Autodesk Fusion 360 part; units mm, degrees
(part 4 of 11)
sketch "Sketch3 (3)" plane through (0, 0, 12.7) normal (0, 0, 1) x (-1, 0, 0)
  arc A0 (-21.5286, -62.8233) -> (-21.5337, -63.9888) centre (0, -63.5) ccw
  arc A1 (-22.9752, -65.6056) -> (-21.5337, -63.9888) centre (-23.1207, -64.0248) ccw
  line L0 (-22.9752, -65.6056) -> (-23.7685, -65.6787)
  spline S0 degree 5 poles (-23.7685, -65.6787) (-23.7824, -65.68) (-23.8102, -65.6829) (-23.8516, -65.6885) (-23.9064, -65.6983) (-23.9746, -65.7135) (-24.0423, -65.731) (-24.1099, -65.7498) (-24.1774, -65.7693) (-24.2448, -65.7894) (-24.3122, -65.81) (-24.3794, -65.8313) (-24.4464, -65.8535) (-24.5132, -65.8769) (-24.5799, -65.9013) (-24.6463, -65.9266) (-24.7126, -65.9529) (-24.7787, -65.9798) (-24.8447, -66.0074) (-24.9105, -66.0355) (-24.9762, -66.0643) (-25.0418, -66.0936) (-25.1072, -66.1236) (-25.1724, -66.1543) (-25.2375, -66.1856) (-25.3025, -66.2176) (-25.3672, -66.2502) (-25.4319, -66.2833) (-25.4964, -66.317) (-25.5607, -66.3513) (-25.6249, -66.386) (-25.6889, -66.4213) (-25.7528, -66.4572) (-25.8165, -66.4935) (-25.8801, -66.5304) (-25.9435, -66.5678) (-26.0067, -66.6057) (-26.0698, -66.6441) (-26.1328, -66.683) (-26.1955, -66.7224) (-26.2582, -66.7622) (-26.3206, -66.8026) (-26.383, -66.8433) (-26.4451, -66.8846) (-26.5071, -66.9263) (-26.5689, -66.9685) (-26.6306, -67.0111) (-26.6921, -67.0541) (-26.7535, -67.0976) (-26.8146, -67.1416) (-26.8757, -67.1859) (-26.9365, -67.2307) (-26.9972, -67.2759) (-27.0577, -67.3215) (-27.1181, -67.3676) (-27.1783, -67.414) (-27.2383, -67.4609) (-27.2981, -67.5082) (-27.3578, -67.5559) (-27.4173, -67.6039) (-27.4767, -67.6524) (-27.5358, -67.7013) (-27.5948, -67.7505) (-27.6536, -67.8002) (-27.7123, -67.8502) (-27.7708, -67.9006) (-27.8291, -67.9514) (-27.8872, -68.0026) (-27.9451, -68.0541) (-28.0029, -68.106) (-28.0605, -68.1583) (-28.1064, -68.2004) (-28.1408, -68.2322) (-28.1636, -68.2534) (-28.1751, -68.264) knots 0 0 0 0 0 0 0.01428571 0.02857143 0.04285714 0.05714286 0.07142857 0.08571429 0.1 0.11428571 0.12857143 0.14285714 0.15714286 0.17142857 0.18571429 0.2 0.21428571 0.22857143 0.24285714 0.25714286 0.27142857 0.28571429 0.3 0.31428571 0.32857143 0.34285714 0.35714286 0.37142857 0.38571429 0.4 0.41428571 0.42857143 0.44285714 0.45714286 0.47142857 0.48571429 0.5 0.51428571 0.52857143 0.54285714 0.55714286 0.57142857 0.58571429 0.6 0.61428571 0.62857143 0.64285714 0.65714286 0.67142857 0.68571429 0.7 0.71428571 0.72857143 0.74285714 0.75714286 0.77142857 0.78571429 0.8 0.81428571 0.82857143 0.84285714 0.85714286 0.87142857 0.88571429 0.9 0.91428571 0.92857143 0.94285714 0.95714286 0.97142857 0.98571429 1 1 1 1 1 1
  arc A2 (-28.1751, -68.264) -> (-27.9081, -69.6374) centre (0, -63.5) ccw
  spline S1 degree 5 poles (-27.9081, -69.6374) (-27.8935, -69.643) (-27.8644, -69.6541) (-27.8206, -69.6707) (-27.7622, -69.6925) (-27.6893, -69.7195) (-27.6163, -69.7459) (-27.5432, -69.772) (-27.4702, -69.7977) (-27.3971, -69.8229) (-27.324, -69.8478) (-27.2509, -69.8722) (-27.1777, -69.8962) (-27.1046, -69.9198) (-27.0314, -69.9429) (-26.9583, -69.9656) (-26.8851, -69.9879) (-26.8119, -70.0097) (-26.7387, -70.0312) (-26.6655, -70.0521) (-26.5923, -70.0727) (-26.5191, -70.0927) (-26.4458, -70.1124) (-26.3726, -70.1316) (-26.2994, -70.1503) (-26.2262, -70.1686) (-26.1531, -70.1864) (-26.0799, -70.2037) (-26.0067, -70.2206) (-25.9336, -70.237) (-25.8605, -70.2529) (-25.7874, -70.2684) (-25.7143, -70.2833) (-25.6412, -70.2978) (-25.5682, -70.3118) (-25.4952, -70.3253) (-25.4223, -70.3383) (-25.3493, -70.3507) (-25.2764, -70.3627) (-25.2036, -70.3742) (-25.1308, -70.3851) (-25.058, -70.3955) (-24.9853, -70.4053) (-24.9127, -70.4146) (-24.8401, -70.4234) (-24.7676, -70.4316) (-24.6951, -70.4392) (-24.6227, -70.4463) (-24.5503, -70.4528) (-24.4781, -70.4587) (-24.4059, -70.4641) (-24.3338, -70.4687) (-24.2618, -70.4727) (-24.1899, -70.4761) (-24.1181, -70.4787) (-24.0464, -70.4807) (-23.9748, -70.4822) (-23.9033, -70.483) (-23.832, -70.4832) (-23.7607, -70.4827) (-23.6896, -70.4814) (-23.6187, -70.479) (-23.548, -70.4756) (-23.4775, -70.4711) (-23.4072, -70.4657) (-23.337, -70.4596) (-23.267, -70.4529) (-23.1971, -70.4458) (-23.1274, -70.4379) (-23.058, -70.4287) (-22.9892, -70.4173) (-22.9346, -70.4058) (-22.8941, -70.3955) (-22.8673, -70.3878) (-22.854, -70.3838) knots -1 -1 -1 -1 -1 -1 -0.98571429 -0.97142857 -0.95714286 -0.94285714 -0.92857143 -0.91428571 -0.9 -0.88571429 -0.87142857 -0.85714286 -0.84285714 -0.82857143 -0.81428571 -0.8 -0.78571429 -0.77142857 -0.75714286 -0.74285714 -0.72857143 -0.71428571 -0.7 -0.68571429 -0.67142857 -0.65714286 -0.64285714 -0.62857143 -0.61428571 -0.6 -0.58571429 -0.57142857 -0.55714286 -0.54285714 -0.52857143 -0.51428571 -0.5 -0.48571429 -0.47142857 -0.45714286 -0.44285714 -0.42857143 -0.41428571 -0.4 -0.38571429 -0.37142857 -0.35714286 -0.34285714 -0.32857143 -0.31428571 -0.3 -0.28571429 -0.27142857 -0.25714286 -0.24285714 -0.22857143 -0.21428571 -0.2 -0.18571429 -0.17142857 -0.15714286 -0.14285714 -0.12857143 -0.11428571 -0.1 -0.08571429 -0.07142857 -0.05714286 -0.04285714 -0.02857143 -0.01428571 0 0 0 0 0 0
  line L1 (-22.854, -70.3838) -> (-22.091, -70.1544)
  arc A3 (-20.1488, -71.1135) -> (-22.091, -70.1544) centre (-21.6338, -71.6746) ccw
  arc A4 (-20.1488, -71.1135) -> (-19.7075, -72.1921) centre (0, -63.5) ccw
  arc A5 (-20.4205, -74.2376) -> (-19.7075, -72.1921) centre (-21.1599, -72.8328) ccw
  line L2 (-20.4205, -74.2376) -> (-21.1255, -74.6087)
  spline S2 degree 5 poles (-21.1255, -74.6087) (-21.1379, -74.6152) (-21.1624, -74.6285) (-21.1985, -74.6495) (-21.2454, -74.6795) (-21.3025, -74.7197) (-21.3585, -74.7617) (-21.4137, -74.805) (-21.4686, -74.8489) (-21.5232, -74.8932) (-21.5775, -74.938) (-21.6314, -74.9834) (-21.6849, -75.0296) (-21.7377, -75.0767) (-21.7899, -75.1248) (-21.8416, -75.1737) (-21.8928, -75.2233) (-21.9435, -75.2734) (-21.9939, -75.3242) (-22.044, -75.3754) (-22.0937, -75.4271) (-22.1431, -75.4793) (-22.192, -75.532) (-22.2405, -75.5853) (-22.2887, -75.6392) (-22.3364, -75.6936) (-22.3838, -75.7485) (-22.4308, -75.8038) (-22.4775, -75.8596) (-22.5239, -75.9159) (-22.5699, -75.9726) (-22.6155, -76.0297) (-22.6608, -76.0872) (-22.7058, -76.1452) (-22.7504, -76.2036) (-22.7946, -76.2624) (-22.8386, -76.3217) (-22.8822, -76.3813) (-22.9254, -76.4413) (-22.9684, -76.5017) (-23.011, -76.5625) (-23.0533, -76.6236) (-23.0952, -76.6852) (-23.1369, -76.7471) (-23.1782, -76.8093) (-23.2192, -76.8719) (-23.2598, -76.9349) (-23.3002, -76.9982) (-23.3402, -77.0619) (-23.3799, -77.1259) (-23.4193, -77.1902) (-23.4584, -77.2549) (-23.4972, -77.3199) (-23.5356, -77.3852) (-23.5738, -77.4508) (-23.6116, -77.5168) (-23.6491, -77.583) (-23.6863, -77.6496) (-23.7232, -77.7165) (-23.7598, -77.7837) (-23.7961, -77.8512) (-23.832, -77.919) (-23.8677, -77.9871) (-23.903, -78.0554) (-23.9381, -78.1241) (-23.9728, -78.193) (-24.0072, -78.2623) (-24.0413, -78.3318) (-24.0752, -78.4016) (-24.1087, -78.4716) (-24.1418, -78.542) (-24.1682, -78.5985) (-24.1878, -78.641) (-24.2008, -78.6693) (-24.2072, -78.6835) knots 0 0 0 0 0 0 0.01428571 0.02857143 0.04285714 0.05714286 0.07142857 0.08571429 0.1 0.11428571 0.12857143 0.14285714 0.15714286 0.17142857 0.18571429 0.2 0.21428571 0.22857143 0.24285714 0.25714286 0.27142857 0.28571429 0.3 0.31428571 0.32857143 0.34285714 0.35714286 0.37142857 0.38571429 0.4 0.41428571 0.42857143 0.44285714 0.45714286 0.47142857 0.48571429 0.5 0.51428571 0.52857143 0.54285714 0.55714286 0.57142857 0.58571429 0.6 0.61428571 0.62857143 0.64285714 0.65714286 0.67142857 0.68571429 0.7 0.71428571 0.72857143 0.74285714 0.75714286 0.77142857 0.78571429 0.8 0.81428571 0.82857143 0.84285714 0.85714286 0.87142857 0.88571429 0.9 0.91428571 0.92857143 0.94285714 0.95714286 0.97142857 0.98571429 1 1 1 1 1 1
  arc A6 (-24.2072, -78.6835) -> (-23.435, -79.8502) centre (0, -63.5) ccw
  spline S3 degree 5 poles (-23.435, -79.8502) (-23.4194, -79.8498) (-23.3882, -79.8489) (-23.3415, -79.8475) (-23.2792, -79.8453) (-23.2015, -79.8422) (-23.1239, -79.8388) (-23.0464, -79.8349) (-22.9691, -79.8307) (-22.8919, -79.8261) (-22.8149, -79.821) (-22.738, -79.8156) (-22.6613, -79.8098) (-22.5846, -79.8036) (-22.5082, -79.7969) (-22.4319, -79.7899) (-22.3558, -79.7825) (-22.2798, -79.7747) (-22.204, -79.7664) (-22.1283, -79.7578) (-22.0528, -79.7488) (-21.9775, -79.7393) (-21.9023, -79.7294) (-21.8274, -79.7191) (-21.7526, -79.7084) (-21.6779, -79.6973) (-21.6035, -79.6857) (-21.5293, -79.6738) (-21.4552, -79.6614) (-21.3814, -79.6485) (-21.3077, -79.6353) (-21.2343, -79.6216) (-21.161, -79.6074) (-21.088, -79.5928) (-21.0152, -79.5778) (-20.9426, -79.5623) (-20.8702, -79.5464) (-20.7981, -79.53) (-20.7261, -79.5132) (-20.6545, -79.4959) (-20.583, -79.4781) (-20.5118, -79.4599) (-20.4409, -79.4412) (-20.3702, -79.4219) (-20.2998, -79.4022) (-20.2296, -79.3821) (-20.1598, -79.3614) (-20.0902, -79.3402) (-20.0208, -79.3186) (-19.9518, -79.2964) (-19.8831, -79.2737) (-19.8147, -79.2504) (-19.7466, -79.2266) (-19.679, -79.2021) (-19.6116, -79.1771) (-19.5446, -79.1515) (-19.4779, -79.1255) (-19.4115, -79.0989) (-19.3455, -79.0718) (-19.2798, -79.044) (-19.2147, -79.0156) (-19.15, -78.9862) (-19.086, -78.956) (-19.0226, -78.9249) (-18.9598, -78.893) (-18.8973, -78.8605) (-18.8351, -78.8276) (-18.7733, -78.7942) (-18.7119, -78.7603) (-18.6513, -78.7252) (-18.5921, -78.6883) (-18.5461, -78.6568) (-18.5126, -78.6318) (-18.4908, -78.6145) (-18.48, -78.6056) knots -1 -1 -1 -1 -1 -1 -0.98571429 -0.97142857 -0.95714286 -0.94285714 -0.92857143 -0.91428571 -0.9 -0.88571429 -0.87142857 -0.85714286 -0.84285714 -0.82857143 -0.81428571 -0.8 -0.78571429 -0.77142857 -0.75714286 -0.74285714 -0.72857143 -0.71428571 -0.7 -0.68571429 -0.67142857 -0.65714286 -0.64285714 -0.62857143 -0.61428571 -0.6 -0.58571429 -0.57142857 -0.55714286 -0.54285714 -0.52857143 -0.51428571 -0.5 -0.48571429 -0.47142857 -0.45714286 -0.44285714 -0.42857143 -0.41428571 -0.4 -0.38571429 -0.37142857 -0.35714286 -0.34285714 -0.32857143 -0.31428571 -0.3 -0.28571429 -0.27142857 -0.25714286 -0.24285714 -0.22857143 -0.21428571 -0.2 -0.18571429 -0.17142857 -0.15714286 -0.14285714 -0.12857143 -0.11428571 -0.1 -0.08571429 -0.07142857 -0.05714286 -0.04285714 -0.02857143 -0.01428571 0 0 0 0 0 0
  line L3 (-18.48, -78.6056) -> (-17.8629, -78.1017)
  arc A7 (-15.7015, -78.2445) -> (-17.8629, -78.1017) centre (-16.8587, -79.3312) ccw
  arc A8 (-15.7015, -78.2445) -> (-14.881, -79.0722) centre (0, -63.5) ccw
  arc A9 (-14.757, -81.2348) -> (-14.881, -79.0722) centre (-15.9777, -80.2199) ccw
  line L4 (-14.757, -81.2348) -> (-15.2663, -81.8475)
  spline S4 degree 5 poles (-15.2663, -81.8475) (-15.2753, -81.8582) (-15.2928, -81.8799) (-15.3181, -81.9131) (-15.35, -81.9588) (-15.3874, -82.0178) (-15.423, -82.078) (-15.4575, -82.1391) (-15.4914, -82.2007) (-15.5248, -82.2625) (-15.5579, -82.3247) (-15.5903, -82.3873) (-15.622, -82.4504) (-15.6528, -82.5142) (-15.6826, -82.5785) (-15.7117, -82.6435) (-15.74, -82.7089) (-15.7677, -82.7747) (-15.7948, -82.8408) (-15.8215, -82.9073) (-15.8476, -82.9741) (-15.8732, -83.0412) (-15.8983, -83.1087) (-15.9227, -83.1765) (-15.9466, -83.2447) (-15.9699, -83.3132) (-15.9927, -83.382) (-16.0149, -83.4512) (-16.0367, -83.5206) (-16.058, -83.5903) (-16.0788, -83.6602) (-16.0991, -83.7305) (-16.1189, -83.801) (-16.1383, -83.8718) (-16.1571, -83.9428) (-16.1755, -84.0141) (-16.1934, -84.0856) (-16.2109, -84.1574) (-16.2279, -84.2294) (-16.2445, -84.3016) (-16.2606, -84.3741) (-16.2762, -84.4468) (-16.2915, -84.5197) (-16.3062, -84.5928) (-16.3206, -84.6661) (-16.3345, -84.7396) (-16.348, -84.8134) (-16.361, -84.8873) (-16.3736, -84.9615) (-16.3858, -85.0358) (-16.3976, -85.1103) (-16.409, -85.185) (-16.4199, -85.2599) (-16.4305, -85.3349) (-16.4406, -85.4102) (-16.4503, -85.4856) (-16.4596, -85.5612) (-16.4685, -85.6369) (-16.477, -85.7128) (-16.4851, -85.7889) (-16.4927, -85.8651) (-16.5, -85.9415) (-16.5069, -86.0181) (-16.5134, -86.0948) (-16.5195, -86.1716) (-16.5252, -86.2486) (-16.5305, -86.3257) (-16.5354, -86.403) (-16.54, -86.4804) (-16.5441, -86.558) (-16.5478, -86.6357) (-16.5505, -86.6979) (-16.5524, -86.7447) (-16.5535, -86.7759) (-16.5541, -86.7915) knots 0 0 0 0 0 0 0.01428571 0.02857143 0.04285714 0.05714286 0.07142857 0.08571429 0.1 0.11428571 0.12857143 0.14285714 0.15714286 0.17142857 0.18571429 0.2 0.21428571 0.22857143 0.24285714 0.25714286 0.27142857 0.28571429 0.3 0.31428571 0.32857143 0.34285714 0.35714286 0.37142857 0.38571429 0.4 0.41428571 0.42857143 0.44285714 0.45714286 0.47142857 0.48571429 0.5 0.51428571 0.52857143 0.54285714 0.55714286 0.57142857 0.58571429 0.6 0.61428571 0.62857143 0.64285714 0.65714286 0.67142857 0.68571429 0.7 0.71428571 0.72857143 0.74285714 0.75714286 0.77142857 0.78571429 0.8 0.81428571 0.82857143 0.84285714 0.85714286 0.87142857 0.88571429 0.9 0.91428571 0.92857143 0.94285714 0.95714286 0.97142857 0.98571429 1 1 1 1 1 1
  arc A10 (-16.5541, -86.7915) -> (-15.3942, -87.5738) centre (0, -63.5) ccw
  spline S5 degree 5 poles (-15.3942, -87.5738) (-15.3799, -87.5675) (-15.3514, -87.5547) (-15.3088, -87.5355) (-15.2521, -87.5097) (-15.1815, -87.4771) (-15.1111, -87.4442) (-15.041, -87.411) (-14.9712, -87.3775) (-14.9017, -87.3437) (-14.8324, -87.3095) (-14.7635, -87.2751) (-14.6948, -87.2404) (-14.6264, -87.2053) (-14.5583, -87.1699) (-14.4905, -87.1342) (-14.423, -87.0983) (-14.3558, -87.0619) (-14.2889, -87.0253) (-14.2223, -86.9884) (-14.156, -86.9511) (-14.09, -86.9136) (-14.0244, -86.8757) (-13.9591, -86.8375) (-13.8941, -86.799) (-13.8294, -86.7601) (-13.765, -86.721) (-13.701, -86.6815) (-13.6374, -86.6417) (-13.574, -86.6016) (-13.5111, -86.5611) (-13.4485, -86.5204) (-13.3862, -86.4793) (-13.3243, -86.4379) (-13.2628, -86.3961) (-13.2016, -86.354) (-13.1409, -86.3116) (-13.0805, -86.2689) (-13.0205, -86.2258) (-12.9609, -86.1824) (-12.9017, -86.1386) (-12.8429, -86.0945) (-12.7845, -86.0501) (-12.7265, -86.0053) (-12.669, -85.9602) (-12.612, -85.9147) (-12.5553, -85.8688) (-12.4991, -85.8226) (-12.4433, -85.7761) (-12.388, -85.7292) (-12.3332, -85.6819) (-12.279, -85.6342) (-12.2252, -85.5862) (-12.172, -85.5377) (-12.1194, -85.4888) (-12.0673, -85.4395) (-12.0156, -85.3899) (-11.9645, -85.34) (-11.9139, -85.2896) (-11.8638, -85.2389) (-11.8145, -85.1876) (-11.766, -85.1358) (-11.7184, -85.0834) (-11.6718, -85.0304) (-11.6259, -84.9769) (-11.5806, -84.9229) (-11.5358, -84.8687) (-11.4914, -84.8142) (-11.4477, -84.7594) (-11.4051, -84.7038) (-11.3645, -84.6471) (-11.3341, -84.6004) (-11.3128, -84.5644) (-11.2992, -84.5401) (-11.2926, -84.5278) knots -1 -1 -1 -1 -1 -1 -0.98571429 -0.97142857 -0.95714286 -0.94285714 -0.92857143 -0.91428571 -0.9 -0.88571429 -0.87142857 -0.85714286 -0.84285714 -0.82857143 -0.81428571 -0.8 -0.78571429 -0.77142857 -0.75714286 -0.74285714 -0.72857143 -0.71428571 -0.7 -0.68571429 -0.67142857 -0.65714286 -0.64285714 -0.62857143 -0.61428571 -0.6 -0.58571429 -0.57142857 -0.55714286 -0.54285714 -0.52857143 -0.51428571 -0.5 -0.48571429 -0.47142857 -0.45714286 -0.44285714 -0.42857143 -0.41428571 -0.4 -0.38571429 -0.37142857 -0.35714286 -0.34285714 -0.32857143 -0.31428571 -0.3 -0.28571429 -0.27142857 -0.25714286 -0.24285714 -0.22857143 -0.21428571 -0.2 -0.18571429 -0.17142857 -0.15714286 -0.14285714 -0.12857143 -0.11428571 -0.1 -0.08571429 -0.07142857 -0.05714286 -0.04285714 -0.02857143 -0.01428571 0 0 0 0 0 0
  line L5 (-11.2926, -84.5278) -> (-10.9153, -83.826)
  arc A11 (-8.8638, -83.1308) -> (-10.9153, -83.826) centre (-9.5171, -84.5777) ccw
  arc A12 (-8.8638, -83.1308) -> (-7.789, -83.5816) centre (0, -63.5) ccw
  arc A13 (-6.8469, -85.5321) -> (-7.789, -83.5816) centre (-8.3631, -85.0616) ccw
  line L6 (-6.8469, -85.5321) -> (-7.083, -86.293)
  spline S6 degree 5 poles (-7.083, -86.293) (-7.0871, -86.3064) (-7.095, -86.3331) (-7.1057, -86.3735) (-7.1177, -86.4279) (-7.1297, -86.4967) (-7.1395, -86.566) (-7.148, -86.6356) (-7.1557, -86.7054) (-7.163, -86.7754) (-7.1697, -86.8455) (-7.1757, -86.9157) (-7.1808, -86.9862) (-7.1849, -87.0569) (-7.1878, -87.1278) (-7.1898, -87.1988) (-7.1909, -87.2701) (-7.1913, -87.3415) (-7.1911, -87.413) (-7.1903, -87.4846) (-7.1889, -87.5563) (-7.1869, -87.6281) (-7.1842, -87.7) (-7.1808, -87.7721) (-7.1768, -87.8442) (-7.1721, -87.9164) (-7.1668, -87.9887) (-7.1609, -88.0611) (-7.1544, -88.1336) (-7.1474, -88.2061) (-7.1399, -88.2787) (-7.1318, -88.3514) (-7.1231, -88.4241) (-7.1139, -88.4969) (-7.1041, -88.5697) (-7.0938, -88.6426) (-7.083, -88.7156) (-7.0717, -88.7886) (-7.0598, -88.8616) (-7.0475, -88.9347) (-7.0346, -89.0078) (-7.0213, -89.0809) (-7.0075, -89.1541) (-6.9931, -89.2273) (-6.9783, -89.3006) (-6.963, -89.3738) (-6.9473, -89.4471) (-6.931, -89.5204) (-6.9143, -89.5937) (-6.8972, -89.6671) (-6.8795, -89.7404) (-6.8614, -89.8138) (-6.8429, -89.8871) (-6.8239, -89.9605) (-6.8045, -90.0339) (-6.7846, -90.1073) (-6.7642, -90.1807) (-6.7435, -90.254) (-6.7223, -90.3274) (-6.7006, -90.4008) (-6.6785, -90.4742) (-6.656, -90.5475) (-6.6331, -90.6209) (-6.6098, -90.6942) (-6.586, -90.7676) (-6.5618, -90.8409) (-6.5372, -90.9142) (-6.5121, -90.9875) (-6.4867, -91.0607) (-6.4608, -91.1339) (-6.4346, -91.2071) (-6.4132, -91.2657) (-6.3971, -91.3096) (-6.3862, -91.3389) (-6.3807, -91.3535) knots 0 0 0 0 0 0 0.01428571 0.02857143 0.04285714 0.05714286 0.07142857 0.08571429 0.1 0.11428571 0.12857143 0.14285714 0.15714286 0.17142857 0.18571429 0.2 0.21428571 0.22857143 0.24285714 0.25714286 0.27142857 0.28571429 0.3 0.31428571 0.32857143 0.34285714 0.35714286 0.37142857 0.38571429 0.4 0.41428571 0.42857143 0.44285714 0.45714286 0.47142857 0.48571429 0.5 0.51428571 0.52857143 0.54285714 0.55714286 0.57142857 0.58571429 0.6 0.61428571 0.62857143 0.64285714 0.65714286 0.67142857 0.68571429 0.7 0.71428571 0.72857143 0.74285714 0.75714286 0.77142857 0.78571429 0.8 0.81428571 0.82857143 0.84285714 0.85714286 0.87142857 0.88571429 0.9 0.91428571 0.92857143 0.94285714 0.95714286 0.97142857 0.98571429 1 1 1 1 1 1
  arc A14 (-6.3807, -91.3535) -> (-5.0097, -91.6324) centre (0, -63.5) ccw
  spline S7 degree 5 poles (-5.0097, -91.6324) (-4.999, -91.6211) (-4.9776, -91.5984) (-4.9455, -91.5643) (-4.903, -91.5188) (-4.8502, -91.4616) (-4.7978, -91.4043) (-4.7457, -91.3468) (-4.6941, -91.2892) (-4.6428, -91.2313) (-4.5919, -91.1733) (-4.5413, -91.1151) (-4.4912, -91.0567) (-4.4414, -90.9981) (-4.392, -90.9394) (-4.343, -90.8805) (-4.2944, -90.8214) (-4.2462, -90.7621) (-4.1984, -90.7027) (-4.1511, -90.6431) (-4.1041, -90.5833) (-4.0575, -90.5233) (-4.0114, -90.4632) (-3.9656, -90.4029) (-3.9203, -90.3425) (-3.8754, -90.2818) (-3.831, -90.221) (-3.7869, -90.1601) (-3.7433, -90.0989) (-3.7002, -90.0376) (-3.6575, -89.9762) (-3.6152, -89.9146) (-3.5735, -89.8528) (-3.5321, -89.7908) (-3.4913, -89.7287) (-3.4509, -89.6664) (-3.411, -89.604) (-3.3715, -89.5414) (-3.3326, -89.4786) (-3.2941, -89.4157) (-3.2561, -89.3526) (-3.2187, -89.2894) (-3.1818, -89.226) (-3.1454, -89.1624) (-3.1095, -89.0987) (-3.0742, -89.0348) (-3.0394, -88.9708) (-3.0052, -88.9066) (-2.9715, -88.8423) (-2.9383, -88.7778) (-2.9058, -88.7131) (-2.8739, -88.6483) (-2.8426, -88.5833) (-2.812, -88.5182) (-2.7821, -88.4529) (-2.7528, -88.3874) (-2.7241, -88.3218) (-2.696, -88.2561) (-2.6684, -88.1902) (-2.6416, -88.1242) (-2.6157, -88.058) (-2.5907, -87.9916) (-2.5668, -87.9249) (-2.544, -87.8581) (-2.5221, -87.7911) (-2.5009, -87.7239) (-2.4802, -87.6567) (-2.4601, -87.5894) (-2.4407, -87.522) (-2.4226, -87.4543) (-2.4068, -87.3864) (-2.3966, -87.3316) (-2.3906, -87.2902) (-2.3874, -87.2625) (-2.386, -87.2486) knots -1 -1 -1 -1 -1 -1 -0.98571429 -0.97142857 -0.95714286 -0.94285714 -0.92857143 -0.91428571 -0.9 -0.88571429 -0.87142857 -0.85714286 -0.84285714 -0.82857143 -0.81428571 -0.8 -0.78571429 -0.77142857 -0.75714286 -0.74285714 -0.72857143 -0.71428571 -0.7 -0.68571429 -0.67142857 -0.65714286 -0.64285714 -0.62857143 -0.61428571 -0.6 -0.58571429 -0.57142857 -0.55714286 -0.54285714 -0.52857143 -0.51428571 -0.5 -0.48571429 -0.47142857 -0.45714286 -0.44285714 -0.42857143 -0.41428571 -0.4 -0.38571429 -0.37142857 -0.35714286 -0.34285714 -0.32857143 -0.31428571 -0.3 -0.28571429 -0.27142857 -0.25714286 -0.24285714 -0.22857143 -0.21428571 -0.2 -0.18571429 -0.17142857 -0.15714286 -0.14285714 -0.12857143 -0.11428571 -0.1 -0.08571429 -0.07142857 -0.05714286 -0.04285714 -0.02857143 -0.01428571 0 0 0 0 0 0
  line L7 (-2.386, -87.2486) -> (-2.306, -86.4559)
  arc A15 (-0.6767, -85.0286) -> (-2.306, -86.4559) centre (-0.7266, -86.6153) ccw
  arc A16 (-0.6767, -85.0286) -> (0.4888, -85.0337) centre (0, -63.5) ccw
  arc A17 (2.1056, -86.4752) -> (0.4888, -85.0337) centre (0.5248, -86.6207) ccw
  line L8 (2.1056, -86.4752) -> (2.1787, -87.2685)
  spline S8 degree 5 poles (2.1787, -87.2685) (2.18, -87.2824) (2.1829, -87.3102) (2.1885, -87.3516) (2.1983, -87.4064) (2.2135, -87.4746) (2.231, -87.5423) (2.2498, -87.6099) (2.2693, -87.6774) (2.2894, -87.7448) (2.31, -87.8122) (2.3313, -87.8794) (2.3535, -87.9464) (2.3769, -88.0132) (2.4013, -88.0799) (2.4266, -88.1463) (2.4529, -88.2126) (2.4798, -88.2787) (2.5074, -88.3447) (2.5355, -88.4105) (2.5643, -88.4762) (2.5936, -88.5418) (2.6236, -88.6072) (2.6543, -88.6724) (2.6856, -88.7375) (2.7176, -88.8025) (2.7502, -88.8672) (2.7833, -88.9319) (2.817, -88.9964) (2.8513, -89.0607) (2.886, -89.1249) (2.9213, -89.1889) (2.9572, -89.2528) (2.9935, -89.3165) (3.0304, -89.3801) (3.0678, -89.4435) (3.1057, -89.5067) (3.1441, -89.5698) (3.183, -89.6328) (3.2224, -89.6955) (3.2622, -89.7582) (3.3026, -89.8206) (3.3433, -89.883) (3.3846, -89.9451) (3.4263, -90.0071) (3.4685, -90.0689) (3.5111, -90.1306) (3.5541, -90.1921) (3.5976, -90.2535) (3.6416, -90.3146) (3.6859, -90.3757) (3.7307, -90.4365) (3.7759, -90.4972) (3.8215, -90.5577) (3.8676, -90.6181) (3.914, -90.6783) (3.9609, -90.7383) (4.0082, -90.7981) (4.0559, -90.8578) (4.1039, -90.9173) (4.1524, -90.9767) (4.2013, -91.0358) (4.2505, -91.0948) (4.3002, -91.1536) (4.3502, -91.2123) (4.4006, -91.2708) (4.4514, -91.3291) (4.5026, -91.3872) (4.5541, -91.4451) (4.606, -91.5029) (4.6583, -91.5605) (4.7004, -91.6064) (4.7322, -91.6408) (4.7534, -91.6636) (4.764, -91.6751) knots 0 0 0 0 0 0 0.01428571 0.02857143 0.04285714 0.05714286 0.07142857 0.08571429 0.1 0.11428571 0.12857143 0.14285714 0.15714286 0.17142857 0.18571429 0.2 0.21428571 0.22857143 0.24285714 0.25714286 0.27142857 0.28571429 0.3 0.31428571 0.32857143 0.34285714 0.35714286 0.37142857 0.38571429 0.4 0.41428571 0.42857143 0.44285714 0.45714286 0.47142857 0.48571429 0.5 0.51428571 0.52857143 0.54285714 0.55714286 0.57142857 0.58571429 0.6 0.61428571 0.62857143 0.64285714 0.65714286 0.67142857 0.68571429 0.7 0.71428571 0.72857143 0.74285714 0.75714286 0.77142857 0.78571429 0.8 0.81428571 0.82857143 0.84285714 0.85714286 0.87142857 0.88571429 0.9 0.91428571 0.92857143 0.94285714 0.95714286 0.97142857 0.98571429 1 1 1 1 1 1
  arc A18 (4.764, -91.6751) -> (6.1374, -91.4081) centre (0, -63.5) ccw
  spline S9 degree 5 poles (6.1374, -91.4081) (6.143, -91.3935) (6.1541, -91.3644) (6.1707, -91.3206) (6.1926, -91.2622) (6.2195, -91.1893) (6.2459, -91.1163) (6.272, -91.0432) (6.2977, -90.9702) (6.3229, -90.8971) (6.3478, -90.824) (6.3722, -90.7509) (6.3962, -90.6778) (6.4198, -90.6046) (6.4429, -90.5314) (6.4656, -90.4583) (6.4879, -90.3851) (6.5097, -90.3119) (6.5312, -90.2387) (6.5521, -90.1655) (6.5727, -90.0923) (6.5927, -90.0191) (6.6124, -89.9458) (6.6316, -89.8726) (6.6503, -89.7994) (6.6686, -89.7262) (6.6864, -89.6531) (6.7037, -89.5799) (6.7206, -89.5067) (6.737, -89.4336) (6.7529, -89.3605) (6.7684, -89.2874) (6.7833, -89.2143) (6.7978, -89.1412) (6.8118, -89.0682) (6.8253, -88.9952) (6.8383, -88.9223) (6.8507, -88.8493) (6.8627, -88.7764) (6.8742, -88.7036) (6.8851, -88.6308) (6.8955, -88.558) (6.9053, -88.4853) (6.9146, -88.4127) (6.9234, -88.3401) (6.9316, -88.2676) (6.9392, -88.1951) (6.9463, -88.1227) (6.9528, -88.0503) (6.9587, -87.9781) (6.9641, -87.9059) (6.9687, -87.8338) (6.9727, -87.7618) (6.9761, -87.6899) (6.9787, -87.6181) (6.9807, -87.5464) (6.9822, -87.4749) (6.983, -87.4034) (6.9832, -87.332) (6.9827, -87.2607) (6.9814, -87.1896) (6.979, -87.1187) (6.9756, -87.048) (6.9711, -86.9775) (6.9657, -86.9072) (6.9596, -86.837) (6.9529, -86.767) (6.9458, -86.6971) (6.9379, -86.6274) (6.9287, -86.558) (6.9173, -86.4892) (6.9058, -86.4346) (6.8955, -86.3941) (6.8878, -86.3673) (6.8838, -86.354) knots -1 -1 -1 -1 -1 -1 -0.98571429 -0.97142857 -0.95714286 -0.94285714 -0.92857143 -0.91428571 -0.9 -0.88571429 -0.87142857 -0.85714286 -0.84285714 -0.82857143 -0.81428571 -0.8 -0.78571429 -0.77142857 -0.75714286 -0.74285714 -0.72857143 -0.71428571 -0.7 -0.68571429 -0.67142857 -0.65714286 -0.64285714 -0.62857143 -0.61428571 -0.6 -0.58571429 -0.57142857 -0.55714286 -0.54285714 -0.52857143 -0.51428571 -0.5 -0.48571429 -0.47142857 -0.45714286 -0.44285714 -0.42857143 -0.41428571 -0.4 -0.38571429 -0.37142857 -0.35714286 -0.34285714 -0.32857143 -0.31428571 -0.3 -0.28571429 -0.27142857 -0.25714286 -0.24285714 -0.22857143 -0.21428571 -0.2 -0.18571429 -0.17142857 -0.15714286 -0.14285714 -0.12857143 -0.11428571 -0.1 -0.08571429 -0.07142857 -0.05714286 -0.04285714 -0.02857143 -0.01428571 0 0 0 0 0 0
  line L9 (6.8838, -86.354) -> (6.6544, -85.591)
  arc A19 (7.6135, -83.6488) -> (6.6544, -85.591) centre (8.1746, -85.1338) ccw
  arc A20 (7.6135, -83.6488) -> (8.6921, -83.2075) centre (0, -63.5) ccw
  arc A21 (10.7376, -83.9205) -> (8.6921, -83.2075) centre (9.3328, -84.6599) ccw
  line L10 (10.7376, -83.9205) -> (11.1087, -84.6255)
  spline S10 degree 5 poles (11.1087, -84.6255) (11.1152, -84.6379) (11.1285, -84.6624) (11.1495, -84.6985) (11.1795, -84.7454) (11.2197, -84.8025) (11.2617, -84.8585) (11.305, -84.9137) (11.3489, -84.9686) (11.3932, -85.0232) (11.438, -85.0775) (11.4834, -85.1314) (11.5296, -85.1849) (11.5767, -85.2377) (11.6248, -85.2899) (11.6737, -85.3416) (11.7233, -85.3928) (11.7734, -85.4435) (11.8242, -85.4939) (11.8754, -85.544) (11.9271, -85.5937) (11.9793, -85.6431) (12.032, -85.692) (12.0853, -85.7405) (12.1392, -85.7887) (12.1936, -85.8364) (12.2485, -85.8838) (12.3038, -85.9308) (12.3596, -85.9775) (12.4159, -86.0239) (12.4726, -86.0699) (12.5297, -86.1155) (12.5872, -86.1608) (12.6452, -86.2058) (12.7036, -86.2504) (12.7624, -86.2946) (12.8217, -86.3386) (12.8813, -86.3822) (12.9413, -86.4254) (13.0017, -86.4684) (13.0625, -86.511) (13.1236, -86.5533) (13.1852, -86.5952) (13.2471, -86.6369) (13.3093, -86.6782) (13.3719, -86.7192) (13.4349, -86.7598) (13.4982, -86.8002) (13.5619, -86.8402) (13.6259, -86.8799) (13.6902, -86.9193) (13.7549, -86.9584) (13.8199, -86.9972) (13.8852, -87.0356) (13.9508, -87.0738) (14.0168, -87.1116) (14.083, -87.1491) (14.1496, -87.1863) (14.2165, -87.2232) (14.2837, -87.2598) (14.3512, -87.2961) (14.419, -87.332) (14.4871, -87.3677) (14.5554, -87.403) (14.6241, -87.4381) (14.693, -87.4728) (14.7623, -87.5072) (14.8318, -87.5413) (14.9016, -87.5752) (14.9716, -87.6087) (15.042, -87.6418) (15.0985, -87.6682) (15.141, -87.6878) (15.1693, -87.7008) (15.1835, -87.7072) knots 0 0 0 0 0 0 0.01428571 0.02857143 0.04285714 0.05714286 0.07142857 0.08571429 0.1 0.11428571 0.12857143 0.14285714 0.15714286 0.17142857 0.18571429 0.2 0.21428571 0.22857143 0.24285714 0.25714286 0.27142857 0.28571429 0.3 0.31428571 0.32857143 0.34285714 0.35714286 0.37142857 0.38571429 0.4 0.41428571 0.42857143 0.44285714 0.45714286 0.47142857 0.48571429 0.5 0.51428571 0.52857143 0.54285714 0.55714286 0.57142857 0.58571429 0.6 0.61428571 0.62857143 0.64285714 0.65714286 0.67142857 0.68571429 0.7 0.71428571 0.72857143 0.74285714 0.75714286 0.77142857 0.78571429 0.8 0.81428571 0.82857143 0.84285714 0.85714286 0.87142857 0.88571429 0.9 0.91428571 0.92857143 0.94285714 0.95714286 0.97142857 0.98571429 1 1 1 1 1 1
  arc A22 (15.1835, -87.7072) -> (16.3502, -86.935) centre (0, -63.5) ccw
  spline S11 degree 5 poles (16.3502, -86.935) (16.3498, -86.9194) (16.3489, -86.8882) (16.3475, -86.8415) (16.3453, -86.7792) (16.3422, -86.7015) (16.3388, -86.6239) (16.3349, -86.5464) (16.3307, -86.4691) (16.3261, -86.3919) (16.321, -86.3149) (16.3156, -86.238) (16.3098, -86.1613) (16.3036, -86.0846) (16.2969, -86.0082) (16.2899, -85.9319) (16.2825, -85.8558) (16.2747, -85.7798) (16.2664, -85.704) (16.2578, -85.6283) (16.2488, -85.5528) (16.2393, -85.4775) (16.2294, -85.4023) (16.2191, -85.3274) (16.2084, -85.2526) (16.1973, -85.1779) (16.1857, -85.1035) (16.1738, -85.0293) (16.1614, -84.9552) (16.1485, -84.8814) (16.1353, -84.8077) (16.1216, -84.7343) (16.1074, -84.661) (16.0928, -84.588) (16.0778, -84.5152) (16.0623, -84.4426) (16.0464, -84.3702) (16.03, -84.2981) (16.0132, -84.2261) (15.9959, -84.1545) (15.9781, -84.083) (15.9599, -84.0118) (15.9412, -83.9409) (15.9219, -83.8702) (15.9022, -83.7998) (15.8821, -83.7296) (15.8614, -83.6598) (15.8402, -83.5902) (15.8186, -83.5208) (15.7964, -83.4518) (15.7737, -83.3831) (15.7504, -83.3147) (15.7266, -83.2466) (15.7021, -83.179) (15.6771, -83.1116) (15.6515, -83.0446) (15.6255, -82.9779) (15.5989, -82.9115) (15.5718, -82.8455) (15.544, -82.7798) (15.5156, -82.7147) (15.4862, -82.65) (15.456, -82.586) (15.4249, -82.5226) (15.393, -82.4598) (15.3605, -82.3973) (15.3276, -82.3351) (15.2942, -82.2733) (15.2603, -82.2119) (15.2252, -82.1513) (15.1883, -82.0921) (15.1568, -82.0461) (15.1318, -82.0126) (15.1145, -81.9908) (15.1056, -81.98) knots -1 -1 -1 -1 -1 -1 -0.98571429 -0.97142857 -0.95714286 -0.94285714 -0.92857143 -0.91428571 -0.9 -0.88571429 -0.87142857 -0.85714286 -0.84285714 -0.82857143 -0.81428571 -0.8 -0.78571429 -0.77142857 -0.75714286 -0.74285714 -0.72857143 -0.71428571 -0.7 -0.68571429 -0.67142857 -0.65714286 -0.64285714 -0.62857143 -0.61428571 -0.6 -0.58571429 -0.57142857 -0.55714286 -0.54285714 -0.52857143 -0.51428571 -0.5 -0.48571429 -0.47142857 -0.45714286 -0.44285714 -0.42857143 -0.41428571 -0.4 -0.38571429 -0.37142857 -0.35714286 -0.34285714 -0.32857143 -0.31428571 -0.3 -0.28571429 -0.27142857 -0.25714286 -0.24285714 -0.22857143 -0.21428571 -0.2 -0.18571429 -0.17142857 -0.15714286 -0.14285714 -0.12857143 -0.11428571 -0.1 -0.08571429 -0.07142857 -0.05714286 -0.04285714 -0.02857143 -0.01428571 0 0 0 0 0 0
  line L11 (15.1056, -81.98) -> (14.6017, -81.3629)
  arc A23 (14.7445, -79.2015) -> (14.6017, -81.3629) centre (15.8312, -80.3587) ccw
  arc A24 (14.7445, -79.2015) -> (15.5722, -78.381) centre (0, -63.5) ccw
  arc A25 (17.7348, -78.257) -> (15.5722, -78.381) centre (16.7199, -79.4777) ccw
  line L12 (17.7348, -78.257) -> (18.3475, -78.7663)
  spline S12 degree 5 poles (18.3475, -78.7663) (18.3582, -78.7753) (18.3799, -78.7928) (18.4131, -78.8181) (18.4588, -78.85) (18.5178, -78.8874) (18.578, -78.923) (18.6391, -78.9575) (18.7007, -78.9914) (18.7625, -79.0248) (18.8247, -79.0579) (18.8873, -79.0903) (18.9504, -79.122) (19.0142, -79.1528) (19.0785, -79.1826) (19.1435, -79.2117) (19.2089, -79.24) (19.2747, -79.2677) (19.3408, -79.2948) (19.4073, -79.3215) (19.4741, -79.3476) (19.5412, -79.3732) (19.6087, -79.3983) (19.6765, -79.4227) (19.7447, -79.4466) (19.8132, -79.4699) (19.882, -79.4927) (19.9512, -79.5149) (20.0206, -79.5367) (20.0903, -79.558) (20.1602, -79.5788) (20.2305, -79.5991) (20.301, -79.6189) (20.3718, -79.6383) (20.4428, -79.6571) (20.5141, -79.6755) (20.5856, -79.6934) (20.6574, -79.7109) (20.7294, -79.7279) (20.8016, -79.7445) (20.8741, -79.7606) (20.9468, -79.7762) (21.0197, -79.7915) (21.0928, -79.8062) (21.1661, -79.8206) (21.2396, -79.8345) (21.3134, -79.848) (21.3873, -79.861) (21.4615, -79.8736) (21.5358, -79.8858) (21.6103, -79.8976) (21.685, -79.909) (21.7599, -79.9199) (21.8349, -79.9305) (21.9102, -79.9406) (21.9856, -79.9503) (22.0612, -79.9596) (22.1369, -79.9685) (22.2128, -79.977) (22.2889, -79.9851) (22.3651, -79.9927) (22.4415, -80) (22.5181, -80.0069) (22.5948, -80.0134) (22.6716, -80.0195) (22.7486, -80.0252) (22.8257, -80.0305) (22.903, -80.0354) (22.9804, -80.04) (23.058, -80.0441) (23.1357, -80.0478) (23.1979, -80.0505) (23.2447, -80.0524) (23.2759, -80.0535) (23.2915, -80.0541) knots 0 0 0 0 0 0 0.01428571 0.02857143 0.04285714 0.05714286 0.07142857 0.08571429 0.1 0.11428571 0.12857143 0.14285714 0.15714286 0.17142857 0.18571429 0.2 0.21428571 0.22857143 0.24285714 0.25714286 0.27142857 0.28571429 0.3 0.31428571 0.32857143 0.34285714 0.35714286 0.37142857 0.38571429 0.4 0.41428571 0.42857143 0.44285714 0.45714286 0.47142857 0.48571429 0.5 0.51428571 0.52857143 0.54285714 0.55714286 0.57142857 0.58571429 0.6 0.61428571 0.62857143 0.64285714 0.65714286 0.67142857 0.68571429 0.7 0.71428571 0.72857143 0.74285714 0.75714286 0.77142857 0.78571429 0.8 0.81428571 0.82857143 0.84285714 0.85714286 0.87142857 0.88571429 0.9 0.91428571 0.92857143 0.94285714 0.95714286 0.97142857 0.98571429 1 1 1 1 1 1
  arc A26 (23.2915, -80.0541) -> (24.0738, -78.8942) centre (0, -63.5) ccw
  spline S13 degree 5 poles (24.0738, -78.8942) (24.0675, -78.8799) (24.0547, -78.8514) (24.0355, -78.8088) (24.0097, -78.7521) (23.9771, -78.6815) (23.9442, -78.6111) (23.911, -78.541) (23.8775, -78.4712) (23.8437, -78.4017) (23.8095, -78.3324) (23.7751, -78.2635) (23.7404, -78.1948) (23.7053, -78.1264) (23.6699, -78.0583) (23.6342, -77.9905) (23.5983, -77.923) (23.5619, -77.8558) (23.5253, -77.7889) (23.4884, -77.7223) (23.4511, -77.656) (23.4136, -77.59) (23.3757, -77.5244) (23.3375, -77.4591) (23.299, -77.3941) (23.2601, -77.3294) (23.221, -77.265) (23.1815, -77.201) (23.1417, -77.1374) (23.1016, -77.074) (23.0611, -77.0111) (23.0204, -76.9485) (22.9793, -76.8862) (22.9379, -76.8243) (22.8961, -76.7628) (22.854, -76.7016) (22.8116, -76.6409) (22.7689, -76.5805) (22.7258, -76.5205) (22.6824, -76.4609) (22.6386, -76.4017) (22.5945, -76.3429) (22.5501, -76.2845) (22.5053, -76.2265) (22.4602, -76.169) (22.4147, -76.112) (22.3688, -76.0553) (22.3226, -75.9991) (22.2761, -75.9433) (22.2292, -75.888) (22.1819, -75.8332) (22.1342, -75.779) (22.0862, -75.7252) (22.0377, -75.672) (21.9888, -75.6194) (21.9395, -75.5673) (21.8899, -75.5156) (21.84, -75.4645) (21.7896, -75.4139) (21.7389, -75.3638) (21.6876, -75.3145) (21.6358, -75.266) (21.5834, -75.2184) (21.5304, -75.1718) (21.4769, -75.1259) (21.4229, -75.0806) (21.3687, -75.0358) (21.3142, -74.9914) (21.2594, -74.9477) (21.2038, -74.9051) (21.1471, -74.8645) (21.1004, -74.8341) (21.0644, -74.8128) (21.0401, -74.7992) (21.0278, -74.7926) knots -1 -1 -1 -1 -1 -1 -0.98571429 -0.97142857 -0.95714286 -0.94285714 -0.92857143 -0.91428571 -0.9 -0.88571429 -0.87142857 -0.85714286 -0.84285714 -0.82857143 -0.81428571 -0.8 -0.78571429 -0.77142857 -0.75714286 -0.74285714 -0.72857143 -0.71428571 -0.7 -0.68571429 -0.67142857 -0.65714286 -0.64285714 -0.62857143 -0.61428571 -0.6 -0.58571429 -0.57142857 -0.55714286 -0.54285714 -0.52857143 -0.51428571 -0.5 -0.48571429 -0.47142857 -0.45714286 -0.44285714 -0.42857143 -0.41428571 -0.4 -0.38571429 -0.37142857 -0.35714286 -0.34285714 -0.32857143 -0.31428571 -0.3 -0.28571429 -0.27142857 -0.25714286 -0.24285714 -0.22857143 -0.21428571 -0.2 -0.18571429 -0.17142857 -0.15714286 -0.14285714 -0.12857143 -0.11428571 -0.1 -0.08571429 -0.07142857 -0.05714286 -0.04285714 -0.02857143 -0.01428571 0 0 0 0 0 0
  line L13 (21.0278, -74.7926) -> (20.326, -74.4153)
  arc A27 (19.6308, -72.3638) -> (20.326, -74.4153) centre (21.0777, -73.0171) ccw
  arc A28 (19.6308, -72.3638) -> (20.0816, -71.289) centre (0, -63.5) ccw
  arc A29 (22.0321, -70.3469) -> (20.0816, -71.289) centre (21.5616, -71.8631) ccw
  line L14 (22.0321, -70.3469) -> (22.793, -70.583)
  spline S14 degree 5 poles (22.793, -70.583) (22.8064, -70.5871) (22.8331, -70.595) (22.8735, -70.6057) (22.9279, -70.6177) (22.9967, -70.6297) (23.066, -70.6395) (23.1356, -70.648) (23.2054, -70.6557) (23.2754, -70.663) (23.3455, -70.6697) (23.4157, -70.6757) (23.4862, -70.6808) (23.5569, -70.6849) (23.6278, -70.6878) (23.6988, -70.6898) (23.7701, -70.6909) (23.8415, -70.6913) (23.913, -70.6911) (23.9846, -70.6903) (24.0563, -70.6889) (24.1281, -70.6869) (24.2, -70.6842) (24.2721, -70.6808) (24.3442, -70.6768) (24.4164, -70.6721) (24.4887, -70.6668) (24.5611, -70.6609) (24.6336, -70.6544) (24.7061, -70.6474) (24.7787, -70.6399) (24.8514, -70.6318) (24.9241, -70.6231) (24.9969, -70.6139) (25.0697, -70.6041) (25.1426, -70.5938) (25.2156, -70.583) (25.2886, -70.5717) (25.3616, -70.5598) (25.4347, -70.5475) (25.5078, -70.5346) (25.5809, -70.5213) (25.6541, -70.5075) (25.7273, -70.4931) (25.8006, -70.4783) (25.8738, -70.463) (25.9471, -70.4473) (26.0204, -70.431) (26.0937, -70.4143) (26.1671, -70.3972) (26.2404, -70.3795) (26.3138, -70.3614) (26.3871, -70.3429) (26.4605, -70.3239) (26.5339, -70.3045) (26.6073, -70.2846) (26.6807, -70.2642) (26.754, -70.2435) (26.8274, -70.2223) (26.9008, -70.2006) (26.9742, -70.1785) (27.0475, -70.156) (27.1209, -70.1331) (27.1942, -70.1098) (27.2676, -70.086) (27.3409, -70.0618) (27.4142, -70.0372) (27.4875, -70.0121) (27.5607, -69.9867) (27.6339, -69.9608) (27.7071, -69.9346) (27.7657, -69.9132) (27.8096, -69.8971) (27.8389, -69.8862) (27.8535, -69.8807) knots 0 0 0 0 0 0 0.01428571 0.02857143 0.04285714 0.05714286 0.07142857 0.08571429 0.1 0.11428571 0.12857143 0.14285714 0.15714286 0.17142857 0.18571429 0.2 0.21428571 0.22857143 0.24285714 0.25714286 0.27142857 0.28571429 0.3 0.31428571 0.32857143 0.34285714 0.35714286 0.37142857 0.38571429 0.4 0.41428571 0.42857143 0.44285714 0.45714286 0.47142857 0.48571429 0.5 0.51428571 0.52857143 0.54285714 0.55714286 0.57142857 0.58571429 0.6 0.61428571 0.62857143 0.64285714 0.65714286 0.67142857 0.68571429 0.7 0.71428571 0.72857143 0.74285714 0.75714286 0.77142857 0.78571429 0.8 0.81428571 0.82857143 0.84285714 0.85714286 0.87142857 0.88571429 0.9 0.91428571 0.92857143 0.94285714 0.95714286 0.97142857 0.98571429 1 1 1 1 1 1
  arc A30 (27.8535, -69.8807) -> (28.1324, -68.5097) centre (0, -63.5) ccw
  spline S15 degree 5 poles (28.1324, -68.5097) (28.1211, -68.499) (28.0984, -68.4776) (28.0643, -68.4455) (28.0188, -68.403) (27.9616, -68.3502) (27.9043, -68.2978) (27.8468, -68.2457) (27.7892, -68.1941) (27.7313, -68.1428) (27.6733, -68.0919) (27.6151, -68.0413) (27.5567, -67.9912) (27.4981, -67.9414) (27.4394, -67.892) (27.3805, -67.843) (27.3214, -67.7944) (27.2621, -67.7462) (27.2027, -67.6984) (27.1431, -67.6511) (27.0833, -67.6041) (27.0233, -67.5575) (26.9632, -67.5114) (26.9029, -67.4656) (26.8425, -67.4203) (26.7818, -67.3754) (26.721, -67.331) (26.6601, -67.2869) (26.5989, -67.2433) (26.5376, -67.2002) (26.4762, -67.1575) (26.4146, -67.1152) (26.3528, -67.0735) (26.2908, -67.0321) (26.2287, -66.9913) (26.1664, -66.9509) (26.104, -66.911) (26.0414, -66.8715) (25.9786, -66.8326) (25.9157, -66.7941) (25.8526, -66.7561) (25.7894, -66.7187) (25.726, -66.6818) (25.6624, -66.6454) (25.5987, -66.6095) (25.5348, -66.5742) (25.4708, -66.5394) (25.4066, -66.5052) (25.3423, -66.4715) (25.2778, -66.4383) (25.2131, -66.4058) (25.1483, -66.3739) (25.0833, -66.3426) (25.0182, -66.312) (24.9529, -66.2821) (24.8874, -66.2528) (24.8218, -66.2241) (24.7561, -66.196) (24.6902, -66.1684) (24.6242, -66.1416) (24.558, -66.1157) (24.4916, -66.0907) (24.4249, -66.0668) (24.3581, -66.044) (24.2911, -66.0221) (24.2239, -66.0009) (24.1567, -65.9802) (24.0894, -65.9601) (24.022, -65.9407) (23.9543, -65.9226) (23.8864, -65.9068) (23.8316, -65.8966) (23.7902, -65.8906) (23.7625, -65.8874) (23.7486, -65.886) knots -1 -1 -1 -1 -1 -1 -0.98571429 -0.97142857 -0.95714286 -0.94285714 -0.92857143 -0.91428571 -0.9 -0.88571429 -0.87142857 -0.85714286 -0.84285714 -0.82857143 -0.81428571 -0.8 -0.78571429 -0.77142857 -0.75714286 -0.74285714 -0.72857143 -0.71428571 -0.7 -0.68571429 -0.67142857 -0.65714286 -0.64285714 -0.62857143 -0.61428571 -0.6 -0.58571429 -0.57142857 -0.55714286 -0.54285714 -0.52857143 -0.51428571 -0.5 -0.48571429 -0.47142857 -0.45714286 -0.44285714 -0.42857143 -0.41428571 -0.4 -0.38571429 -0.37142857 -0.35714286 -0.34285714 -0.32857143 -0.31428571 -0.3 -0.28571429 -0.27142857 -0.25714286 -0.24285714 -0.22857143 -0.21428571 -0.2 -0.18571429 -0.17142857 -0.15714286 -0.14285714 -0.12857143 -0.11428571 -0.1 -0.08571429 -0.07142857 -0.05714286 -0.04285714 -0.02857143 -0.01428571 0 0 0 0 0 0
  line L15 (23.7486, -65.886) -> (22.9559, -65.806)
  arc A31 (21.5286, -64.1767) -> (22.9559, -65.806) centre (23.1153, -64.2266) ccw
  arc A32 (21.5286, -64.1767) -> (21.5337, -63.0112) centre (0, -63.5) ccw
  arc A33 (22.9752, -61.3944) -> (21.5337, -63.0112) centre (23.1207, -62.9752) ccw
  line L16 (22.9752, -61.3944) -> (23.7685, -61.3213)
  spline S16 degree 5 poles (23.7685, -61.3213) (23.7824, -61.32) (23.8102, -61.3171) (23.8516, -61.3115) (23.9065, -61.3017) (23.9746, -61.2865) (24.0423, -61.269) (24.1099, -61.2502) (24.1774, -61.2307) (24.2448, -61.2106) (24.3122, -61.19) (24.3794, -61.1687) (24.4464, -61.1465) (24.5132, -61.1231) (24.5799, -61.0987) (24.6463, -61.0734) (24.7126, -61.0471) (24.7787, -61.0202) (24.8447, -60.9926) (24.9105, -60.9645) (24.9762, -60.9357) (25.0418, -60.9064) (25.1072, -60.8764) (25.1724, -60.8457) (25.2375, -60.8144) (25.3025, -60.7824) (25.3672, -60.7498) (25.4319, -60.7167) (25.4964, -60.683) (25.5607, -60.6487) (25.6249, -60.614) (25.6889, -60.5787) (25.7528, -60.5428) (25.8165, -60.5065) (25.8801, -60.4696) (25.9435, -60.4322) (26.0067, -60.3943) (26.0698, -60.3559) (26.1328, -60.317) (26.1955, -60.2776) (26.2582, -60.2378) (26.3206, -60.1974) (26.383, -60.1567) (26.4451, -60.1154) (26.5071, -60.0737) (26.5689, -60.0315) (26.6306, -59.9889) (26.6921, -59.9459) (26.7535, -59.9024) (26.8146, -59.8584) (26.8757, -59.8141) (26.9365, -59.7693) (26.9972, -59.7241) (27.0577, -59.6785) (27.1181, -59.6324) (27.1783, -59.586) (27.2383, -59.5391) (27.2981, -59.4918) (27.3578, -59.4441) (27.4173, -59.3961) (27.4767, -59.3476) (27.5358, -59.2987) (27.5948, -59.2495) (27.6536, -59.1998) (27.7123, -59.1498) (27.7708, -59.0994) (27.8291, -59.0486) (27.8872, -58.9974) (27.9451, -58.9459) (28.0029, -58.894) (28.0605, -58.8417) (28.1064, -58.7996) (28.1408, -58.7678) (28.1636, -58.7466) (28.1751, -58.736) knots 0 0 0 0 0 0 0.01428571 0.02857143 0.04285714 0.05714286 0.07142857 0.08571429 0.1 0.11428571 0.12857143 0.14285714 0.15714286 0.17142857 0.18571429 0.2 0.21428571 0.22857143 0.24285714 0.25714286 0.27142857 0.28571429 0.3 0.31428571 0.32857143 0.34285714 0.35714286 0.37142857 0.38571429 0.4 0.41428571 0.42857143 0.44285714 0.45714286 0.47142857 0.48571429 0.5 0.51428571 0.52857143 0.54285714 0.55714286 0.57142857 0.58571429 0.6 0.61428571 0.62857143 0.64285714 0.65714286 0.67142857 0.68571429 0.7 0.71428571 0.72857143 0.74285714 0.75714286 0.77142857 0.78571429 0.8 0.81428571 0.82857143 0.84285714 0.85714286 0.87142857 0.88571429 0.9 0.91428571 0.92857143 0.94285714 0.95714286 0.97142857 0.98571429 1 1 1 1 1 1
  arc A34 (28.1751, -58.736) -> (27.9081, -57.3626) centre (0, -63.5) ccw
  spline S17 degree 5 poles (27.9081, -57.3626) (27.8935, -57.357) (27.8644, -57.3459) (27.8206, -57.3293) (27.7622, -57.3074) (27.6893, -57.2805) (27.6163, -57.2541) (27.5432, -57.228) (27.4702, -57.2023) (27.3971, -57.1771) (27.324, -57.1522) (27.2509, -57.1278) (27.1778, -57.1038) (27.1046, -57.0802) (27.0314, -57.0571) (26.9583, -57.0344) (26.8851, -57.0121) (26.8119, -56.9903) (26.7387, -56.9688) (26.6655, -56.9479) (26.5923, -56.9273) (26.5191, -56.9073) (26.4458, -56.8876) (26.3726, -56.8684) (26.2994, -56.8497) (26.2262, -56.8314) (26.1531, -56.8136) (26.0799, -56.7963) (26.0067, -56.7794) (25.9336, -56.763) (25.8605, -56.7471) (25.7874, -56.7316) (25.7143, -56.7167) (25.6412, -56.7022) (25.5682, -56.6882) (25.4952, -56.6747) (25.4223, -56.6617) (25.3493, -56.6493) (25.2764, -56.6373) (25.2036, -56.6258) (25.1308, -56.6149) (25.058, -56.6045) (24.9853, -56.5947) (24.9127, -56.5854) (24.8401, -56.5766) (24.7676, -56.5684) (24.6951, -56.5608) (24.6227, -56.5537) (24.5503, -56.5472) (24.4781, -56.5413) (24.4059, -56.5359) (24.3338, -56.5313) (24.2618, -56.5273) (24.1899, -56.5239) (24.1181, -56.5213) (24.0464, -56.5193) (23.9749, -56.5178) (23.9034, -56.517) (23.832, -56.5168) (23.7607, -56.5173) (23.6896, -56.5186) (23.6187, -56.521) (23.548, -56.5244) (23.4775, -56.5289) (23.4072, -56.5343) (23.337, -56.5404) (23.267, -56.5471) (23.1971, -56.5542) (23.1274, -56.5621) (23.058, -56.5713) (22.9892, -56.5827) (22.9346, -56.5942) (22.8941, -56.6045) (22.8673, -56.6122) (22.854, -56.6162) knots -1 -1 -1 -1 -1 -1 -0.98571429 -0.97142857 -0.95714286 -0.94285714 -0.92857143 -0.91428571 -0.9 -0.88571429 -0.87142857 -0.85714286 -0.84285714 -0.82857143 -0.81428571 -0.8 -0.78571429 -0.77142857 -0.75714286 -0.74285714 -0.72857143 -0.71428571 -0.7 -0.68571429 -0.67142857 -0.65714286 -0.64285714 -0.62857143 -0.61428571 -0.6 -0.58571429 -0.57142857 -0.55714286 -0.54285714 -0.52857143 -0.51428571 -0.5 -0.48571429 -0.47142857 -0.45714286 -0.44285714 -0.42857143 -0.41428571 -0.4 -0.38571429 -0.37142857 -0.35714286 -0.34285714 -0.32857143 -0.31428571 -0.3 -0.28571429 -0.27142857 -0.25714286 -0.24285714 -0.22857143 -0.21428571 -0.2 -0.18571429 -0.17142857 -0.15714286 -0.14285714 -0.12857143 -0.11428571 -0.1 -0.08571429 -0.07142857 -0.05714286 -0.04285714 -0.02857143 -0.01428571 0 0 0 0 0 0
  line L17 (22.854, -56.6162) -> (22.091, -56.8456)
  arc A35 (20.1488, -55.8865) -> (22.091, -56.8456) centre (21.6338, -55.3254) ccw
  arc A36 (20.1488, -55.8865) -> (19.7075, -54.8079) centre (0, -63.5) ccw
  arc A37 (20.4205, -52.7624) -> (19.7075, -54.8079) centre (21.1599, -54.1672) ccw
  line L18 (20.4205, -52.7624) -> (21.1255, -52.3913)
  spline S18 degree 5 poles (21.1255, -52.3913) (21.1379, -52.3848) (21.1624, -52.3715) (21.1985, -52.3505) (21.2454, -52.3205) (21.3025, -52.2803) (21.3585, -52.2383) (21.4137, -52.195) (21.4686, -52.1511) (21.5232, -52.1068) (21.5775, -52.062) (21.6314, -52.0166) (21.6849, -51.9704) (21.7377, -51.9233) (21.7899, -51.8752) (21.8416, -51.8263) (21.8928, -51.7767) (21.9435, -51.7266) (21.9939, -51.6758) (22.044, -51.6246) (22.0937, -51.5729) (22.1431, -51.5207) (22.192, -51.468) (22.2405, -51.4147) (22.2887, -51.3608) (22.3364, -51.3064) (22.3838, -51.2515) (22.4308, -51.1962) (22.4775, -51.1404) (22.5239, -51.0841) (22.5699, -51.0274) (22.6155, -50.9703) (22.6608, -50.9128) (22.7058, -50.8548) (22.7504, -50.7964) (22.7946, -50.7376) (22.8386, -50.6783) (22.8822, -50.6187) (22.9254, -50.5587) (22.9684, -50.4983) (23.011, -50.4375) (23.0533, -50.3764) (23.0952, -50.3148) (23.1369, -50.2529) (23.1782, -50.1907) (23.2192, -50.1281) (23.2598, -50.0651) (23.3002, -50.0018) (23.3402, -49.9381) (23.3799, -49.8741) (23.4193, -49.8098) (23.4584, -49.7451) (23.4972, -49.6801) (23.5356, -49.6148) (23.5738, -49.5492) (23.6116, -49.4832) (23.6491, -49.417) (23.6863, -49.3504) (23.7232, -49.2835) (23.7598, -49.2163) (23.7961, -49.1488) (23.832, -49.081) (23.8677, -49.0129) (23.903, -48.9446) (23.9381, -48.8759) (23.9728, -48.807) (24.0072, -48.7377) (24.0413, -48.6682) (24.0752, -48.5984) (24.1087, -48.5284) (24.1418, -48.458) (24.1682, -48.4015) (24.1878, -48.359) (24.2008, -48.3307) (24.2072, -48.3165) knots 0 0 0 0 0 0 0.01428571 0.02857143 0.04285714 0.05714286 0.07142857 0.08571429 0.1 0.11428571 0.12857143 0.14285714 0.15714286 0.17142857 0.18571429 0.2 0.21428571 0.22857143 0.24285714 0.25714286 0.27142857 0.28571429 0.3 0.31428571 0.32857143 0.34285714 0.35714286 0.37142857 0.38571429 0.4 0.41428571 0.42857143 0.44285714 0.45714286 0.47142857 0.48571429 0.5 0.51428571 0.52857143 0.54285714 0.55714286 0.57142857 0.58571429 0.6 0.61428571 0.62857143 0.64285714 0.65714286 0.67142857 0.68571429 0.7 0.71428571 0.72857143 0.74285714 0.75714286 0.77142857 0.78571429 0.8 0.81428571 0.82857143 0.84285714 0.85714286 0.87142857 0.88571429 0.9 0.91428571 0.92857143 0.94285714 0.95714286 0.97142857 0.98571429 1 1 1 1 1 1
  arc A38 (24.2072, -48.3165) -> (23.435, -47.1498) centre (0, -63.5) ccw